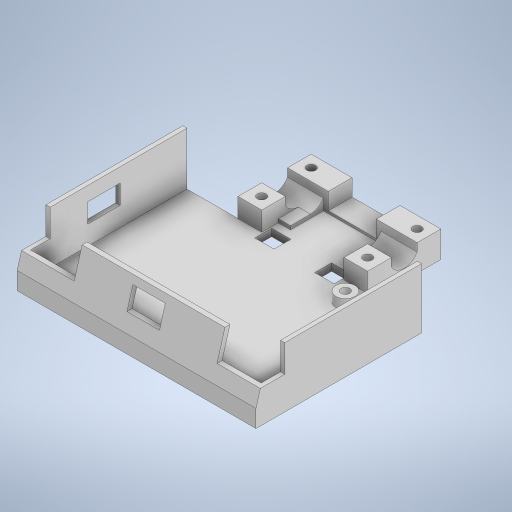
# Autodesk Inventor part: Součást1
Saved by Autodesk Inventor 2024 (Build 280153000, 153)
## iProperties
Created: 2023-09-06
Part Number: Součást1
Material: Všeobecné
Document SubType Name: Modeling
Designer: Simak
Density: 1 g/cm^3
Appearance: Výchozí
Author: Simak
Autodesk Inventor part; units mm, degrees
ref_plane "YZ Plane" through (0, 0, 0) normal (1, 0, 0) x (0, 1, 0)
ref_plane "XZ Plane" through (0, 0, 0) normal (0, 1, 0) x (-1, 0, 0)
ref_plane "XY Plane" through (0, 0, 0) normal (0, 0, 1) x (1, 0, 0)
sketch "Náčrt1" plane through (0, 0, 0) normal (0, 1, 0) x (-1, 0, 0)
  line L0 (49.75, -19.25) -> (49.75, 49.75)
  line L1 (49.75, 49.75) -> (-49.75, 49.75)
  line L2 (-49.75, 49.75) -> (-49.75, -19.25)
  line L3 (-49.75, -19.25) -> (-27.25, -19.25)
  line L4 (-27.25, -19.25) -> (-27.25, -49.75)
  line L5 (-27.25, -49.75) -> (26.75, -49.75)
  line L6 (26.75, -49.75) -> (26.75, -19.25)
  line L7 (26.75, -19.25) -> (49.75, -19.25)
  point P0 (0, 0)
  dimension "d0" = 30.5
  dimension "d1" = 99.5
  dimension "d2" = 22.5
  dimension "d3" = 99.5
  dimension "d4" = 54
  dimension "d5" = 49.75
  dimension "d6" = 49.75
  constraints: 16 end point, 6 perpendicular, 2 vertical, 1 parallel
  measures "d0" distance of L3.end L4.end
  measures "d1" distance of L0.end L1.end
  measures "d2" distance of L2.end L3.end
  measures "d3" distance between parallel lines of L1 L5
  measures "d4" distance of L4.end L5.end
  measures "d5" horizontal distance of L1.end point (0, 0)
  measures "d6" distance from line of point (0, 0) L1
extrude "Vysunutí1" add sketch "Náčrt1" along normal blind 3
sketch "Náčrt2" plane through (27.25, 0, -19.25) normal (1, 0, 0) x (0, 0, -1)
  line L0 (30.5, 3) -> (0, 3)
  line L1 (0, 3) -> (0, 11)
  line L2 (0, 11) -> (9.875, 11)
  line L3 (9.875, 11) -> (9.875, 7.646)
  arc A0 (9.875, 7.646) -> (20.625, 7.646) centre (15.25, 10.582835) ccw
  line L4 (20.625, 7.646) -> (20.625, 11)
  line L5 (20.625, 11) -> (30.5, 11)
  line L6 (30.5, 11) -> (30.5, 3)
  line L7 (0, 0) -> (30.5, 0)
  point P0 (-19.25, 0)
  dimension "d9" = 6.125
  dimension "d10" = 11
  dimension "d11" = 9.875
  dimension "d12" = 3.354
  constraints: 12 end point, 3 perpendicular, 2 equal length, 2 point on circle, 2 point on line, 1 centre point, 1 parallel, 1 vertical
  measures "d9" radius of A0
  measures "d10" distance between parallel lines of L5 L7
  measures "d11" distance of L4.end L5.end
  measures "d12" distance of L4.start L4.end
extrude "Vysunutí2" add sketch "Náčrt2" against normal up to surface (54 mm away)
sketch "Náčrt3" plane through (27.25, 3, -19.25) normal (0, 0, 1) x (1, 0, 0)
  line L0 (0, 8) -> (-54, 8) projected
  line L1 (-39, 8) -> (-39, 0)
  line L2 (-15, 8) -> (-15, 0)
  line L3 (-77, 0) -> (22.5, 0) projected
  line L4 (0, 8) -> (0, 0) projected
  line L5 (-54, 8) -> (-54, 0) projected
  line L6 (-15, 4) -> (0, 4)
  line L7 (-39, 4) -> (-54, 4)
  point P0 (-27.25, -3)
  dimension "d24" = 24
  constraints: 8 end point, 4 midpoint, 4 point on line, 2 vertical, 1 collinear
  measures "d24" distance between parallel lines of L1 L2
extrude "Vysunutí3" cut sketch "Náčrt3" against normal up to surface (20.625 mm away) contours L2 L3 L1 L0
sketch "Náčrt4" plane through (-26.75, 3, -19.25) normal (0, 0, 1) x (1, 0, 0)
  line L0 (0, 1.457835) -> (15, 1.457835)
  line L1 (39, 1.457835) -> (54, 1.457835)
  line L2 (9.875, 1.457835) -> (9.875, 8)
  line L3 (54, 8) -> (0, 8)
  line L4 (0, 8) -> (0, 0)
  line L5 (44.125, 8) -> (44.125, 1.457835)
  line L6 (54, 8) -> (54, 0)
  line L7 (15, 0) -> (15, 8)
  line L8 (39, 8) -> (39, 0)
  point P0 (26.75, -3)
  dimension "d20" = 9.875
  dimension "d21" = 9.875
  constraints: 4 end point, 4 point on line, 2 vertical
  measures "d20" distance between parallel lines of L4 L2
  measures "d21" distance between parallel lines of L6 L5
extrude "Vysunutí4" cut sketch "Náčrt4" against normal up to next contours L2 L3 L7 L0 | L8 L3 L5 L1
sketch "Náčrt5" plane through (-26.75, 3, -19.25) normal (0, 0, 1) x (1, 0, 0)
  line L0 (9.875, 1.457835) -> (9.875, 0)
  line L1 (15, 0) -> (0, 0)
  line L2 (44.125, 1.457835) -> (44.125, 0)
  line L3 (54, 0) -> (39, 0)
  line L4 (15, 1.457835) -> (9.875, 1.457835)
  line L5 (15, 0) -> (15, 1.457835)
  line L6 (-23, 0) -> (76.5, 0)
  line L7 (39, 1.457835) -> (39, 0)
  line L8 (44.125, 1.457835) -> (39, 1.457835)
  point P0 (26.75, -3)
  constraints: 4 end point, 2 coincident, 2 point on line, 1 parallel, 1 vertical
extrude "Vysunutí5" cut sketch "Náčrt5" against normal blind 6.875
sketch "Náčrt6" plane through (27.25, 7.646, -39.875) normal (0, 0, 1) x (1, 0, 0)
  line L0 (0, 3.354) -> (-54, 3.354) projected
  line L1 (-37, 3.354) -> (-37, -3.646)
  line L2 (-37, -3.646) -> (-17, -3.646)
  line L3 (-17, -3.646) -> (-17, 3.354)
  line L4 (-77, -4.646) -> (22.5, -4.646) projected
  line L5 (0, 3.354) -> (0, 0) projected
  line L6 (-17, -0.146) -> (0, -0.146) construction
  line L7 (-37, -0.146) -> (-54, -0.146) construction
  line L8 (-54, -7.646) -> (-54, 3.354) projected
  point P0 (-27.25, -7.646)
  dimension "d27" = 1
  dimension "d35" = 20
  constraints: 10 end point, 4 point on line, 2 horizontal, 2 midpoint, 2 perpendicular, 1 collinear, 1 vertical
  measures "d27" distance between parallel lines of L4 L2
  measures "d35" distance of L1.end L2.end
extrude "Vysunutí6" cut sketch "Náčrt6" against normal up to next
sketch "Náčrt7" plane through (-26.75, 11, -19.25) normal (0, 1, 0) x (1, 0, 0)
  circle A0 centre (4.9375, 4.9375) radius 1.85
  circle A1 centre (4.9375, 25.5625) radius 1.85
  circle A2 centre (49.0625, 25.5625) radius 1.85
  circle A3 centre (49.0625, 4.9375) radius 1.85
  line L0 (76.5, 0) -> (54, 0) projected
  line L1 (49.0625, 4.9375) -> (54, 0) construction
  line L2 (54, 0) -> (44.125, 0) projected
  line L3 (44.125, 0) -> (49.0625, 4.9375) construction
  line L4 (54, 9.875) -> (49.0625, 4.9375) construction
  line L5 (9.875, 0) -> (9.875, 6.875) projected
  line L6 (4.9375, 4.9375) -> (9.875, 0) construction
  line L7 (0, 30.5) -> (0, 0) projected
  line L8 (0, 0) -> (4.9375, 4.9375) construction
  line L9 (4.9375, 4.9375) -> (0, 9.875) construction
  line L10 (0, 20.625) -> (4.9375, 25.5625) construction
  line L11 (4.9375, 25.5625) -> (0, 30.5) construction
  line L12 (54, 0) -> (54, 30.5) projected
  line L13 (54, 20.625) -> (49.0625, 25.5625) construction
  line L14 (49.0625, 25.5625) -> (54, 30.5) construction
  point P0 (26.75, -19.25)
  dimension "d36" = 3.7
  constraints: 20 end point, 12 equal length, 4 centre point, 3 equal radius, 1 coincident
  measures "d36" diameter of A1
extrude "Vysunutí7" cut sketch "Náčrt7" against normal through all
sketch "Náčrt8" plane through (0, 3, 0) normal (0, 1, 0) x (1, 0, 0)
  circle A0 centre (-44.06, -43.75) radius 4
  circle A1 centre (-44.06, -43.75) radius 1.85
  circle A2 centre (43.94, -43.75) radius 4
  circle A3 centre (43.94, -43.75) radius 1.85
  line L0 (-44.06, -43.75) -> (-49.75, -43.75) construction
  line L1 (-49.75, 19.25) -> (-49.75, -49.75) projected
  line L2 (43.94, -43.75) -> (49.75, -43.75) construction
  line L3 (49.75, -49.75) -> (49.75, 19.25) projected
  circle A4 centre (25.71, 11.53) radius 1.85
  circle A5 centre (25.71, 11.53) radius 4
  line L4 (-49.75, -49.75) -> (49.75, -49.75) projected
  point P0 (0, 0)
  dimension "d39" = 88
  dimension "d40" = 61.28
  dimension "d41" = 75.46
  dimension "d42" = 6
  dimension "d43" = 8
  dimension "d44" = 3.7
  dimension "d60" = 5.81
  constraints: 6 centre point, 4 end point, 4 equal radius, 3 coincident, 3 point on line, 2 horizontal
  measures "d39" distance of A2.centre A0.centre
  measures "d40" distance from line of A4.centre L4
  measures "d41" distance from line of L1 A4.centre
  measures "d42" distance from line of L4 A2.centre
  measures "d43" diameter of A2
  measures "d44" diameter of A3
  measures "d60" distance of L2.start L2.end
extrude "Vysunutí8" cut sketch "Náčrt8" along normal through all both and the other way through all contours A1 | A3 | A4
extrude "Vysunutí9" add sketch "Náčrt8" along normal blind 4
sketch "Náčrt9" plane through (0, 0, 0) normal (0, -1, 0) x (1, 0, 0)
  circle A0 centre (-44.06, 43.75) radius 1.85
  line L0 (-41.235, 45.381015) -> (-41.235, 42.118985)
  line L1 (-41.235, 42.118985) -> (-44.06, 40.487971)
  line L2 (-44.06, 40.487971) -> (-46.885, 42.118985)
  line L3 (-46.885, 42.118985) -> (-46.885, 45.381015)
  line L4 (-46.885, 45.381015) -> (-44.06, 47.012029)
  line L5 (-44.06, 47.012029) -> (-41.235, 45.381015)
  circle A1 centre (43.94, 43.75) radius 1.85
  line L6 (46.765, 45.381015) -> (46.765, 42.118985)
  line L7 (46.765, 42.118985) -> (43.94, 40.487971)
  line L8 (43.94, 40.487971) -> (41.115, 42.118985)
  line L9 (41.115, 42.118985) -> (41.115, 45.381015)
  line L10 (41.115, 45.381015) -> (43.94, 47.012029)
  line L11 (43.94, 47.012029) -> (46.765, 45.381015)
  circle A2 centre (25.71, -11.53) radius 1.85
  line L12 (28.535, -9.898985) -> (28.535, -13.161015)
  line L13 (28.535, -13.161015) -> (25.71, -14.792029)
  line L14 (25.71, -14.792029) -> (22.885, -13.161015)
  line L15 (22.885, -13.161015) -> (22.885, -9.898985)
  line L16 (22.885, -9.898985) -> (25.71, -8.267971)
  line L17 (25.71, -8.267971) -> (28.535, -9.898985)
  circle A3 centre (-21.8125, -24.1875) radius 1.85
  line L18 (-18.9875, -22.556485) -> (-18.9875, -25.818515)
  line L19 (-18.9875, -25.818515) -> (-21.8125, -27.449529)
  line L20 (-21.8125, -27.449529) -> (-24.6375, -25.818515)
  line L21 (-24.6375, -25.818515) -> (-24.6375, -22.556485)
  line L22 (-24.6375, -22.556485) -> (-21.8125, -20.925471)
  line L23 (-21.8125, -20.925471) -> (-18.9875, -22.556485)
  circle A4 centre (22.3125, -24.1875) radius 1.85
  line L24 (19.4875, -25.818515) -> (19.4875, -22.556485)
  line L25 (19.4875, -22.556485) -> (22.3125, -20.925471)
  line L26 (22.3125, -20.925471) -> (25.1375, -22.556485)
  line L27 (25.1375, -22.556485) -> (25.1375, -25.818515)
  line L28 (25.1375, -25.818515) -> (22.3125, -27.449529)
  line L29 (22.3125, -27.449529) -> (19.4875, -25.818515)
  circle A5 centre (22.3125, -44.8125) radius 1.85
  line L30 (19.4875, -43.181485) -> (22.3125, -41.550471)
  line L31 (22.3125, -41.550471) -> (25.1375, -43.181485)
  line L32 (25.1375, -43.181485) -> (25.1375, -46.443515)
  line L33 (25.1375, -46.443515) -> (22.3125, -48.074529)
  line L34 (22.3125, -48.074529) -> (19.4875, -46.443515)
  line L35 (19.4875, -46.443515) -> (19.4875, -43.181485)
  line L36 (-18.9875, -43.181485) -> (-18.9875, -46.443515)
  line L37 (-18.9875, -46.443515) -> (-21.8125, -48.074529)
  line L38 (-21.8125, -48.074529) -> (-24.6375, -46.443515)
  line L39 (-24.6375, -46.443515) -> (-24.6375, -43.181485)
  line L40 (-24.6375, -43.181485) -> (-21.8125, -41.550471)
  line L41 (-21.8125, -41.550471) -> (-18.9875, -43.181485)
  circle A6 centre (-21.8125, -44.8125) radius 1.85
  point P0 (0, 0)
  dimension "d50" = 5.65
  constraints: 84 end point, 7 coincident, 7 vertical, 6 equal length, 91 other
  measures "d50" distance between parallel lines of L3 L0
extrude "Vysunutí10" cut sketch "Náčrt9" against normal blind 4 contours A0 | L0 L1 L2 L3 L4 L5 | A1 | L6 L7 L8 L9 L10 L11 | A2 | L12 L13 L14 L15 L16 L17
extrude "Vysunutí11" cut sketch "Náčrt9" against normal blind 4 contours A3 | L18 L19 L20 L21 L22 L23 | A4 | L24 L25 L26 L27 L28 L29 | A5 | L30 L31 L32 L33 L34 L35 | L36 L37 L38 L39 L40 L41 | A6
sketch "Náčrt10" plane through (49.75, 0, 49.75) normal (1, 0, 0) x (0, 0, -1)
  line L0 (0, 0) -> (7.142857, 25)
  line L1 (10, 7) -> (2, 7)
  line L2 (5.062826, 25) -> (0, 7.28011)
  line L3 (0, 0) -> (69, 0)
  line L4 (0, 0) -> (0, 7.28011)
  line L5 (5.062826, 25) -> (7.142857, 25)
  line L6 (2, 3) -> (2, 7)
  line L7 (0, 3) -> (69, 3)
  point P0 (49.75, 0)
  point P1 (0.857143, 3)
  dimension "d55" = 2
  dimension "d56" = 25
  constraints: 8 end point, 1 horizontal, 1 horizontal alignment, 1 parallel, 1 point on line, 1 vertical, 1 vertical alignment
  measures "d55" distance between parallel lines of L2 L0
  measures "d56" distance from line of L3 L2.start
extrude "Vysunutí12" add sketch "Náčrt10" against normal up to surface (99.5 mm away)
sketch "Náčrt11" plane through (49.75, 0, 49.75) normal (1, 0, 0) x (0, 0, -1)
  line L0 (10, 7) -> (2, 7)
  line L1 (2.25, 7) -> (2.25, 9)
  line L2 (2.25, 9) -> (10, 9)
  line L3 (10, 9) -> (10, 7)
  line L4 (2.25, 9) -> (2.808441, 9.829544)
  line L5 (2, 7) -> (7.142857, 25)
  point P0 (49.75, 0)
  point P1 (2.25, 7.875)
  dimension "d61" = 2
  dimension "d62" = 0.25
  dimension "d65" = 1
  constraints: 8 end point, 2 perpendicular, 2 point on line, 1 vertical
  measures "d61" distance of L2.end L0.start
  measures "d62" distance from line of L0.end L1
  measures "d65" distance of L1.end L4.end
extrude "Vysunutí13" cut sketch "Náčrt11" against normal through all contours L1 L2 L5 | L2 L4 L5
sketch "Náčrt12" plane through (0, 3, 0) normal (0, 1, 0) x (1, 0, 0)
  line L0 (-49.75, 19.25) -> (-49.75, -47.75)
  line L1 (-26.75, 19.25) -> (-49.75, 19.25)
  line L2 (49.75, 19.25) -> (27.25, 19.25)
  line L3 (49.75, -47.75) -> (49.75, 19.25)
  line L4 (43.94, -47.75) -> (49.75, -47.75)
  line L5 (-49.75, -47.75) -> (-44.06, -47.75)
  line L6 (-48, -47.75) -> (-48, 19.25)
  line L7 (48, -47.75) -> (48, 19.25)
  line L8 (49.75, -42.607143) -> (-49.75, -42.607143)
  point P0 (0, 0)
  point P1 (-48, -42.607143)
  point P2 (48, -42.607143)
  dimension "d66" = 1.75
  dimension "d67" = 1.75
  constraints: 4 end point, 4 point on line, 1 perpendicular, 1 vertical
  measures "d66" distance between parallel lines of L6 L0
  measures "d67" distance between parallel lines of L3 L7
extrude "Vysunutí14" add sketch "Náčrt12" along normal up to surface (22 mm away) contours L1 L6 L8 L0 | L3 L8 L7 L2
sketch "Náčrt13" plane through (48, 3, 42.607143) normal (0, 0, 1) x (1, 0, 0)
  line L0 (1.75, 22) -> (0, 22) projected
  line L1 (0, 0) -> (0, 22) projected
  line L2 (1.75, 0) -> (0, 0) projected
  line L3 (1.75, 0) -> (1.75, 22) projected
  line L4 (-96, 22) -> (-97.75, 22) projected
  line L5 (-97.75, 0) -> (-97.75, 22) projected
  line L6 (-96, 0) -> (-97.75, 0) projected
  line L7 (-96, 0) -> (-96, 22) projected
  point P0 (-48, -3)
extrude "Vysunutí15" add sketch "Náčrt13" along normal up to next
sketch "Náčrt14" plane through (0, 7, 0) normal (0, 1, 0) x (1, 0, 0)
  arc A0 (-44.06, -47.75) -> (-48, -43.059783) centre (-44.06, -43.75) ccw
  arc A1 (-48, -44.440217) -> (-44.06, -47.75) centre (-44.06, -43.75) ccw
  line L0 (-48, -43.059783) -> (-48, -44.440217)
  line L1 (-48, -43.059783) -> (-48, -44.440217)
  arc A2 (-48, -44.440217) -> (-44.06, -47.75) centre (-44.06, -43.75) ccw
  arc A3 (-44.06, -47.75) -> (-48, -43.059783) centre (-44.06, -43.75) ccw
  circle A4 centre (-44.06, -43.75) radius 1.85
  circle A5 centre (43.94, -43.75) radius 4
  circle A6 centre (-44.06, -43.75) radius 4
  circle A7 centre (43.94, -43.75) radius 1.85
  line L2 (48, -42.607143) -> (-48, -42.607143)
  line L3 (42.09, -43.75) -> (42.09, -42.607143)
  circle A8 centre (43.94, -43.75) radius 1.85
  line L4 (45.79, -43.75) -> (45.79, -42.607143)
  line L5 (-45.91, -43.75) -> (-45.91, -42.607143)
  line L6 (-42.21, -43.75) -> (-42.21, -42.607143)
  point P0 (0, 0)
  point P1 (43.94, -47.75)
  point P2 (-42.605223, -42.607143)
  point P3 (-45.514777, -42.607143)
  point P4 (45.394777, -42.607143)
  point P5 (42.485223, -42.607143)
  constraints: 8 end point, 4 perpendicular, 4 point on circle, 4 point on line, 3 tangent, 1 centre point, 1 coincident, 1 concentric, 1 horizontal alignment, 1 vertical, 1 vertical alignment
extrude "Vysunutí16" cut sketch "Náčrt14" along normal up to next contours L6 A4 L2 | L2 A4 L5 | L2 A4 | A4 L2 | L4 A7 L2 | L2 A7 L3 | L2 A7 | A7 L2
sketch "Náčrt15" plane through (0, 0, 0) normal (0, -1, 0) x (1, 0, 0)
  line L0 (20.75, 38.25) -> (13.75, 38.25)
  line L1 (13.75, 38.25) -> (13.75, 46.25)
  line L2 (13.75, 46.25) -> (20.75, 46.25)
  line L3 (20.75, 46.25) -> (20.75, 38.25)
  line L4 (-17.25, 38.25) -> (-24.25, 38.25)
  line L5 (-24.25, 38.25) -> (-24.25, 46.25)
  line L6 (-24.25, 46.25) -> (-17.25, 46.25)
  line L7 (-17.25, 46.25) -> (-17.25, 38.25)
  line L8 (-49.75, 49.75) -> (49.75, 49.75) projected
  line L9 (49.75, 49.75) -> (49.75, -19.25) projected
  line L10 (-49.75, -19.25) -> (-49.75, 49.75) projected
  line L11 (8.75, -22.75) -> (16.75, -22.75)
  line L12 (16.75, -22.75) -> (16.75, -15.75)
  line L13 (16.75, -15.75) -> (8.75, -15.75)
  line L14 (8.75, -15.75) -> (8.75, -22.75)
  line L15 (-16.25, -22.75) -> (-8.25, -22.75)
  line L16 (-8.25, -22.75) -> (-8.25, -15.75)
  line L17 (-8.25, -15.75) -> (-16.25, -15.75)
  line L18 (-16.25, -15.75) -> (-16.25, -22.75)
  line L19 (49.75, -19.25) -> (27.25, -19.25) projected
  line L20 (-26.75, -49.75) -> (-26.75, -19.25) projected
  line L21 (27.25, -19.25) -> (27.25, -49.75) projected
  point P0 (0, 0)
  point P1 (-12.25, -22.75)
  point P2 (12.75, -22.75)
  dimension "d74" = 8
  dimension "d75" = 3.5
  dimension "d76" = 7
  dimension "d77" = 29
  dimension "d78" = 25.5
  dimension "d79" = 3.5
  dimension "d80" = 10.5
  dimension "d81" = 10.5
  constraints: 32 end point, 8 parallel, 6 equal length, 4 horizontal, 4 perpendicular, 2 midpoint, 2 point on line, 1 horizontal alignment
  measures "d74" distance of L0.end L1.end
  measures "d75" distance between parallel lines of L8 L2
  measures "d76" distance of L0.start L0.end
  measures "d77" distance between parallel lines of L9 L3
  measures "d78" distance between parallel lines of L10 L5
  measures "d79" distance between parallel lines of L11 L19
  measures "d80" distance between parallel lines of L20 L18
  measures "d81" distance between parallel lines of L12 L21
extrude "Vysunutí17" cut sketch "Náčrt15" against normal up to surface (3 mm away)
sketch "Náčrt16" plane through (-49.75, 0, -19.25) normal (-1, 0, 0) x (0, 0, 1)
  line L0 (30.4, 16.63) -> (38.9, 16.63)
  line L1 (38.9, 16.63) -> (38.9, 13.63)
  line L2 (38.9, 13.63) -> (30.4, 13.63)
  line L3 (30.4, 13.63) -> (30.4, 16.63)
  line L4 (41.4, 19.13) -> (27.9, 19.13)
  line L5 (27.9, 19.13) -> (27.9, 11.13)
  line L6 (27.9, 11.13) -> (41.4, 11.13)
  line L7 (41.4, 11.13) -> (41.4, 19.13)
  line L8 (0, 0) -> (69, 0) projected
  line L9 (0, 0) -> (0, 25) projected
  point P0 (19.25, 0)
  dimension "d84" = 3
  dimension "d85" = 8.5
  dimension "d86" = 2.5
  dimension "d87" = 13.63
  dimension "d91" = 30.4
  constraints: 16 end point, 4 parallel, 2 perpendicular, 1 horizontal, 3 other
  measures "d84" distance of L0.end L1.end
  measures "d85" distance of L0.start L0.end
  measures "d86" distance between parallel lines of L0 L4
  measures "d87" distance between parallel lines of L8 L2
  measures "d91" distance between parallel lines of L9 L3
extrude "Vysunutí18" cut sketch "Náčrt16" against normal up to surface (1.75 mm away) contours L0 L1 L2 L3 | L7 L6 L5 L4
sketch "Náčrt17" plane through (-49.75, 0, 49.75) normal (0, 0, 1) x (1, 0, 0)
  line L0 (44, 22.1) -> (44, 13.6)
  line L1 (0, 25) -> (0, 7.28011)
  line L2 (57.5, 22.1) -> (57.5, 13.6)
  line L3 (99.5, 25) -> (99.5, 7.28011)
  line L4 (44, 13.6) -> (57.5, 13.6)
  line L5 (57.5, 22.1) -> (44, 22.1)
  line L6 (92.094944, 25) -> (7.285056, 25)
  point P0 (49.75, 0)
  dimension "d92" = 44
  dimension "d93" = 42
  dimension "d94" = 8.5
  dimension "d95" = 2.9
  constraints: 8 end point, 2 vertical, 1 horizontal, 1 parallel
  measures "d92" distance between parallel lines of L1 L0
  measures "d93" distance between parallel lines of L3 L2
  measures "d94" distance of L2.start L2.end
  measures "d95" distance between parallel lines of L5 L6
extrude "Vysunutí19" cut sketch "Náčrt17" against normal up to next
sketch "Náčrt18" plane through (-49.75, 0, 49.75) normal (0, 0, 1) x (1, 0, 0)
  line L0 (99.5, 0) -> (99.5, 25)
  line L1 (81.5, 25) -> (99.5, 25)
  line L2 (99.5, 25) -> (99.5, 13.6)
  line L3 (99.5, 13.6) -> (81.5, 13.6)
  line L4 (81.5, 13.6) -> (81.5, 25)
  line L5 (0, 19.13) -> (0, 11.13)
  line L6 (22, 25) -> (0, 25)
  line L7 (0, 25) -> (0, 13.6)
  line L8 (0, 13.6) -> (22, 13.6)
  line L9 (22, 13.6) -> (22, 25)
  line L10 (57.5, 22.1) -> (57.5, 13.6)
  line L11 (44, 22.1) -> (57.5, 22.1)
  line L12 (92.094944, 25) -> (7.285056, 25)
  point P0 (49.75, 0)
  dimension "d101" = 18
  dimension "d102" = 22
  constraints: 16 end point, 4 parallel, 4 point on line, 2 horizontal, 2 horizontal alignment, 2 perpendicular
  measures "d101" distance of L1.start L1.end
  measures "d102" distance of L6.start L6.end
extrude "Vysunutí20" cut sketch "Náčrt18" against normal blind 12
